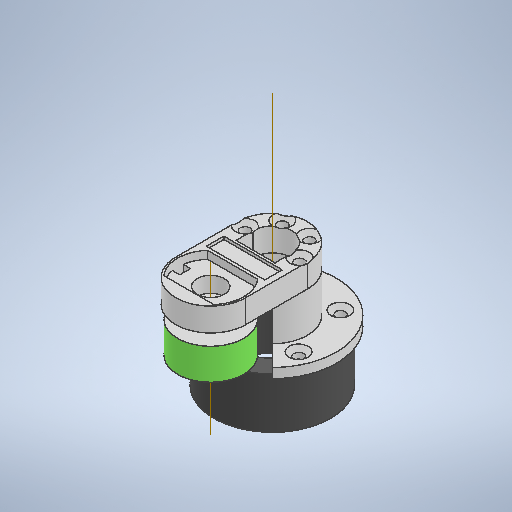
# Autodesk Inventor part: Collective_Angle_Reader
Saved by Autodesk Inventor 2026.2 (Build 302298000, 298)
## iProperties
Created: 2026-03-05
Part Number: Collective_Angle_Reader
Material: Generic
Document SubType Name: Modeling
Designer: Paco Ariel
Density: 1 g/cm^3
Appearance: Default
Author: Paco Ariel
Autodesk Inventor part; units mm, degrees
ref_plane "YZ Plane" through (0, 0, 0) normal (1, 0, 0) x (0, 1, 0)
ref_plane "XY Plane" through (0, 0, 0) normal (0, 0, 1) x (1, 0, 0)
sketch "Sketch3" plane through (0, 0, 0) normal (0, 1, 0) x (-1, 0, 0)
  line L0 (0, 0) -> (0, -15.8205)
  dimension "d15" = 15.8205
  constraints: 2 end point, 1 vertical
  measures "d15" distance of L0.start L0.end
ref_plane "Work Plane3" through (0, 5.8, 0) normal (0, 1, 0) x (-1, 0, 0)
ref_plane "Work Plane2" through (0, 9.8, 0) normal (0, 1, 0) x (-1, 0, 0)
sketch "Sketch1" plane through (0, 5.8, 0) normal (0, 1, 0) x (-1, 0, 0)
  circle A0 centre (0, 0) radius 3.5
  arc A1 (9, 0) -> (-9, 0) centre (0, 0) ccw
  line L0 (9, 0) -> (9, -15.8205)
  line L1 (-9, 0) -> (-9, -15.8205)
  arc A2 (-9, -15.8205) -> (9, -15.8205) centre (0, -15.8205) ccw
  dimension "d3" = 7
  dimension "d4" = 18
  constraints: 4 end point, 4 point on circle, 3 centre point, 3 coincident, 3 tangent, 2 vertical
  measures "d3" diameter of A0
  measures "d4" diameter of A1
extrude "Extrusion1" add sketch "Sketch1" along normal blind 6
sketch "Sketch2" plane through (0, 11.8, 0) normal (0, 1, 0) x (1, 0, 0)
  line L0 (7.5, 10.875) -> (-7.5, 10.875)
  line L1 (-7.5, 10.875) -> (-7.5, 6.375)
  line L2 (-7.5, 6.375) -> (7.5, 6.375)
  line L3 (7.5, 6.375) -> (7.5, 10.875)
  line L4 (7.5, 10.875) -> (-7.5, 6.375) construction
  line L5 (-7.5, 10.875) -> (7.5, 6.375) construction
  line L6 (6.4391, -5.625) -> (-6.4391, -5.625)
  line L7 (-6.4391, 5.625) -> (6.4391, 5.625)
  line L8 (7.5349, -4.0407) -> (7.5, -4.022) construction
  arc A0 (-6.4391, 5.625) -> (-6.4391, -5.625) centre (0, 0) ccw
  arc A1 (6.4391, -5.625) -> (6.4391, 5.625) centre (0, 0) ccw
  line L9 (-6.5654, 1.4) -> (-8.4346, 1.4)
  line L10 (-8.4346, -1.4) -> (-6.5654, -1.4)
  line L11 (-6.5654, -1.4) -> (-6.5654, 1.4)
  point P0 (0, 0)
  point P1 (0, 8.625)
  point P2 (-7.5, -1.4)
  point P3 (-8.4346, 1.4)
  dimension "d10" = 4.5
  dimension "d12" = 15
  dimension "d13" = 11.25
  dimension "d14" = 8.625
  dimension "d22" = 7.5
  dimension "d23" = 2.8
  constraints: 24 end point, 6 point on circle, 4 parallel, 3 horizontal, 2 centre point, 2 midpoint, 1 coincident, 1 perpendicular, 1 point on line
  measures "d10" distance of L1.end L0.end
  measures "d12" distance of L0.start L0.end
  measures "d13" distance between parallel lines of L6 L7
  measures "d14" distance of point (0, 8.625) point (0, 0)
  measures "d22" horizontal distance of point (-7.5, -1.4) point (0, 0)
  measures "d23" distance between parallel lines of L9 L10
extrude "Extrusion2" cut sketch "Sketch2" against normal blind 2 contours L6 A0 L10 L11 L9 L7 A1 | A0 L9 L11 L10
extrude "Extrusion3" cut sketch "Sketch2" against normal blind 0.75 contours L3 L2 L1 L0
extrude "Extrusion4" cut sketch "Sketch2" against normal blind 4.5 contours A0 L9 L11 L10
ref_plane "Work Plane4" through (0, -7, 0) normal (0, 1, 0) x (-1, 0, 0)
sketch "Sketch4" plane through (0, -7, 0) normal (0, 1, 0) x (-1, 0, 0)
  circle A0 centre (0, -15.8205) radius 10
  circle A1 centre (0, -15.8205) radius 14.95
  point P0 (0, 0)
  dimension "d27" = 20
  dimension "d28" = 29.9
  constraints: 2 centre point, 2 coincident
  measures "d27" diameter of A0
  measures "d28" diameter of A1
extrude "Extrusion5" add sketch "Sketch4" against normal blind 13 separate body
sketch "Sketch5" plane through (0, 11.8, 0) normal (0, 1, 0) x (1, 0, 0)
  line L0 (0, 0) -> (0, 11.5)
  line L1 (-5, 11.5) -> (5, 11.5)
  line L2 (-5, 13.5) -> (5, 13.5)
  line L3 (5, 13.5) -> (5, 11.5)
  line L4 (9, 0) -> (9, 15.8205) projected
  line L5 (-5, 13.5) -> (-5, 11.5)
  arc A0 (5, 15.8205) -> (-5, 15.8205) centre (0, 15.8205) ccw
  line L6 (-5, 15.8205) -> (-5, 13.5)
  line L7 (5, 15.8205) -> (5, 13.5)
  point P0 (-4.4289, 13.5)
  point P1 (4.4289, 13.5)
  dimension "d31" = 11.5
  dimension "d32" = 2
  dimension "d73" = 10
  dimension "d74" = 10
  constraints: 14 end point, 2 parallel, 2 point on circle, 2 point on line, 2 tangent, 2 vertical, 1 centre point, 1 collinear, 1 horizontal, 1 midpoint
  measures "d31" distance of L0.start L0.end
  measures "d32" distance between parallel lines of L1 L2
  measures "d73" diameter of A0
  measures "d74" distance between parallel lines of L3 L5
extrude "Extrusion6" cut sketch "Sketch5" against normal through all bodies 1
sketch "Sketch6" plane through (0, 2.5, 0) normal (0, 1, 0) x (-1, 0, 0)
  circle A0 centre (0, 0) radius 8.5
  dimension "d35" = 17
  constraints: 1 centre point, 1 coincident
  measures "d35" diameter of A0
extrude "Extrusion7" add sketch "Sketch6" against normal blind 8 separate body
sketch "Sketch7" plane through (0, -7, -15.8205) normal (0, 1, 0) x (1, 0, 0)
  line L0 (-3.5355, -3.5355) -> (-11.6319, -11.6319)
  line L1 (0, 0) -> (14.95, 0) construction
  line L2 (3.5355, -3.5355) -> (11.6319, -11.6319)
  line L3 (0, 0) -> (14.95, 0) construction
  arc A0 (11.6319, -11.6319) -> (-11.6319, -11.6319) centre (0, 0) ccw
  arc A1 (3.5355, -3.5355) -> (-3.5355, -3.5355) centre (0, 0) ccw
  line L4 (-5, 0) -> (-5, -5.8122)
  line L5 (-5, -4.3205) -> (-5, 0) projected
  line L6 (5, 0) -> (5, -4.3205) projected
  line L7 (5, 0) -> (5, -5.9836)
  point P0 (0, -15.8205)
  point P1 (-5, -5)
  point P2 (5, -5)
  dimension "d38" = 135
  dimension "d39" = 45
  dimension "d57" = 5
  dimension "d58" = 16.45
  constraints: 12 end point, 6 point on circle, 2 centre point, 2 coincident, 2 collinear, 2 horizontal, 1 point on line
  measures "d38" angle of L0 L1
  measures "d39" angle of L2 L3
  measures "d57" radius of A1
  measures "d58" radius of A0
sketch "Sketch9" plane through (0, -7, -15.8205) normal (0, 1, 0) x (1, 0, 0)
  circle A0 centre (0, 0) radius 12.475
  line L0 (0, 0) -> (35.4408, -14.6801)
  line L1 (7.0711, -7.0711) -> (11.6319, -11.6319) projected
  line L2 (0, 0) -> (-30.1447, -12.4864)
  line L3 (-7.0711, -7.0711) -> (-10.5712, -10.5712) projected
  point P0 (0, -15.8205)
  point P1 (7.0711, -7.0711)
  point P2 (14.95, 0)
  point P3 (11.5254, -4.774)
  point P4 (-11.5254, -4.774)
  point P5 (7.5943, 9.8971)
  point P6 (-7.5943, 9.8971)
  point P7 (-11.5254, -4.774)
  point P8 (11.6319, -11.6319)
  dimension "d41" = 24.95
  dimension "d42" = 22.5
  dimension "d43" = 22.5
  dimension "d46" = 225
  constraints: 4 end point, 2 point on circle, 2 point on line, 1 centre point, 5 other
  measures "d41" diameter of A0
  measures "d42" angle to the sketch x axis of L0
  measures "d43" angle of L3 L2
hole "Hole1" at (11.5254, -7, -11.0465) at (7.5943, -7, -25.7176) at (-7.5943, -7, -25.7176) at (-11.5254, -7, -11.0465) direction (0, -1, 0) diameter 3.2 depth 4 tip angle 118 bodies 2
extrude "Extrusion8" add sketch "Sketch7" along normal blind 2.5 separate body contours L0 A0 L2 L7 L6 A1 L4
hole "Hole2" at (11.5254, -7, -11.0465) at (7.5943, -7, -25.7176) at (-7.5943, -7, -25.7176) at (-11.5254, -7, -11.0465) direction (0, 1, 0) diameter 2.5 depth 2.5 tip angle 118 bodies 4
chamfer "Chamfer1" distance 1.2 distance2 1 4 edges at (11.5254, -4.5, -9.7965) (7.5943, -4.5, -24.4676) (-7.5943, -4.5, -24.4676) (-11.5254, -4.5, -9.7965) measured on face at (7.5943, -4.5, -23.9676) measured on face at (-7.5943, -4.5, -23.9676) measured on face at (11.5254, -4.5, -9.2965) measured on face at (-11.5254, -4.5, -9.2965)
sketch "Sketch10" plane through (0, -4.5, -15.8205) normal (0, 1, 0) x (1, 0, 0)
  arc A0 (9, 0) -> (-9, 0) centre (0, 0) ccw projected
  circle A1 centre (0, 0) radius 9
  arc A2 (5, 0) -> (-5, 0) centre (0, 0) ccw projected
  line L0 (5, -5) -> (11.6319, -11.6319) projected
  line L1 (-11.6319, -11.6319) -> (-5, -5) projected
  line L2 (5, 0) -> (5, -4.3205) projected
  line L3 (5, 0) -> (5, -5) projected
  line L4 (-5, -5) -> (-5, 0) projected
  point P0 (0, -15.8205)
  point P1 (-3.5355, -3.5355)
  point P2 (3.5355, -3.5355)
  point P3 (6.364, -6.364)
  point P4 (9, 0)
  point P5 (-9, 0)
  point P6 (-6.364, -6.364)
  constraints: 1 centre point, 1 coincident, 1 concentric
extrude "Extrusion9" add sketch "Sketch10" along normal up to surface (10.3 mm away) contours A1 L0 L3 L2 A2 L4 L1 A0 bodies 4
sketch "Sketch11" plane through (0, 11.8, 0) normal (0, 1, 0) x (1, 0, 0)
  arc A0 (5, 15.8205) -> (-5, 15.8205) centre (0, 15.8205) ccw projected
  arc A1 (9, 15.8205) -> (-9, 15.8205) centre (0, 15.8205) ccw projected
  line L0 (-9, 15.8205) -> (-5, 15.8205)
  line L1 (5, 15.8205) -> (9, 15.8205)
  line L2 (-4.5, 23.6147) -> (-2.5, 20.1506)
  line L3 (4.5, 23.6147) -> (2.5, 20.1506)
  line L4 (9, 15.8205) -> (5, 15.8205)
  point P0 (0, 0)
  point P1 (-7, 15.8205)
  point P2 (-3.5, 21.8827)
  point P3 (3.5, 21.8827)
  point P4 (7, 15.8205)
  dimension "d78" = 180
  constraints: 10 end point, 4 midpoint, 1 collinear, 1 horizontal, 10 other
hole "Hole3" at (7, 11.8, -15.8205) at (3.5, 11.8, -21.8827) at (-3.5, 11.8, -21.8827) at (-7, 11.8, -15.8205) direction (0, -1, 0) diameter 2.5 depth 6 tip angle 118 bodies 1
chamfer "Chamfer2" distance 1.2 distance2 1 4 edges at (-7, 11.8, -17.0705) (-3.5, 11.8, -23.1327) (3.5, 11.8, -23.1327) (7, 11.8, -17.0705) measured on face at (3.5, 11.8, -23.6327) measured on face at (-7, 11.8, -17.5705) measured on face at (-3.5, 11.8, -23.6327) measured on face at (7, 11.8, -17.5705)
hole "Hole4" at (-7, 11.8, -15.8205) at (-3.5, 11.8, -21.8827) at (3.5, 11.8, -21.8827) at (7, 11.8, -15.8205) direction (0, -1, 0) diameter 2.5 depth 13 tip angle 118 bodies 4
hole "Hole5" at (7, 11.8, -15.8205) at (3.5, 11.8, -21.8827) at (-3.5, 11.8, -21.8827) at (-7, 11.8, -15.8205) direction (0, -1, 0) diameter 3.2 depth 10 tip angle 175 bodies 4
ref_plane "Work Plane1" through (0, 2.5, 0) normal (0, 1, 0) x (-1, 0, 0)
body "Solid1"
body "Solid2"
body "Solid3"
body "Solid5"
